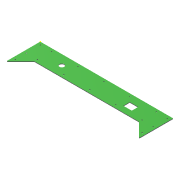
# Autodesk Inventor part: Acrylic Front Panel - No Graphics
Saved by Autodesk Inventor 2017 (Build 210142000, 142)
## iProperties
Created: 2016-07-11
Part Number: Acrylic Front Panel - No Graphics
Material: Generic
Document SubType Name: Modeling
Designer: joshm
Density: 1 g/cm^3
Appearance: Default
Author: joshm
Autodesk Inventor part; units mm, degrees
(part 1 of 2)
ref_plane "YZ Plane" through (0, 0, 0) normal (1, 0, 0) x (0, 1, 0)
ref_plane "XZ Plane" through (0, 0, 0) normal (0, 1, 0) x (-1, 0, 0)
ref_plane "XY Plane" through (0, 0, 0) normal (0, 0, 1) x (1, 0, 0)
sketch "Sketch1" plane through (0, 0, 0) normal (0, 0, 1) x (1, 0, 0)
  line L0 (659.9602, -164.404) -> (660, -164)
  line L1 (660, -164) -> (660, 0)
  line L2 (660, 0) -> (0, 0)
  line L3 (0, 0) -> (0, -164)
  line L4 (0, -164) -> (0.0398, -164.404)
  line L5 (0.0398, -164.404) -> (0.1577, -164.7926)
  line L6 (0.1577, -164.7926) -> (0.349, -165.1506)
  line L7 (0.349, -165.1506) -> (0.6066, -165.4645)
  line L8 (0.6066, -165.4645) -> (0.9204, -165.722)
  line L9 (0.9204, -165.722) -> (1.2785, -165.9134)
  line L10 (1.2785, -165.9134) -> (1.667, -166.0313)
  line L11 (1.667, -166.0313) -> (2.0711, -166.0711)
  line L12 (2.0711, -166.0711) -> (2.4751, -166.0313)
  line L13 (2.4751, -166.0313) -> (2.8636, -165.9134)
  line L14 (2.8636, -165.9134) -> (3.2217, -165.722)
  line L15 (3.2217, -165.722) -> (3.5355, -165.4645)
  line L16 (3.5355, -165.4645) -> (70, -99)
  line L17 (70, -99) -> (590, -99)
  line L18 (590, -99) -> (656.4645, -165.4645)
  line L19 (656.4645, -165.4645) -> (656.7783, -165.722)
  line L20 (656.7783, -165.722) -> (657.1364, -165.9134)
  line L21 (657.1364, -165.9134) -> (657.5249, -166.0313)
  line L22 (657.5249, -166.0313) -> (657.9289, -166.0711)
  line L23 (657.9289, -166.0711) -> (658.333, -166.0313)
  line L24 (658.333, -166.0313) -> (658.7215, -165.9134)
  line L25 (658.7215, -165.9134) -> (659.0796, -165.722)
  line L26 (659.0796, -165.722) -> (659.3934, -165.4645)
  line L27 (659.3934, -165.4645) -> (659.651, -165.1506)
  line L28 (659.651, -165.1506) -> (659.8423, -164.7926)
  line L29 (659.8423, -164.7926) -> (659.9602, -164.404)
  line L30 (590.6522, -86.4341) -> (590, -86.52)
  line L31 (590, -86.52) -> (589.3478, -86.4341)
  line L32 (589.3478, -86.4341) -> (588.74, -86.1824)
  line L33 (588.74, -86.1824) -> (588.2181, -85.7819)
  line L34 (588.2181, -85.7819) -> (587.8176, -85.26)
  line L35 (587.8176, -85.26) -> (587.5659, -84.6522)
  line L36 (587.5659, -84.6522) -> (587.48, -84)
  line L37 (587.48, -84) -> (587.5659, -83.3478)
  line L38 (587.5659, -83.3478) -> (587.8176, -82.74)
  line L39 (587.8176, -82.74) -> (588.2181, -82.2181)
  line L40 (588.2181, -82.2181) -> (588.74, -81.8176)
  line L41 (588.74, -81.8176) -> (589.3478, -81.5659)
  line L42 (589.3478, -81.5659) -> (590, -81.48)
  line L43 (590, -81.48) -> (590.6522, -81.5659)
  line L44 (590.6522, -81.5659) -> (591.26, -81.8176)
  line L45 (591.26, -81.8176) -> (591.7819, -82.2181)
  line L46 (591.7819, -82.2181) -> (592.1824, -82.74)
  line L47 (592.1824, -82.74) -> (592.4341, -83.3478)
  line L48 (592.4341, -83.3478) -> (592.52, -84)
  line L49 (592.52, -84) -> (592.4341, -84.6522)
  line L50 (592.4341, -84.6522) -> (592.1824, -85.26)
  line L51 (592.1824, -85.26) -> (591.7819, -85.7819)
  line L52 (591.7819, -85.7819) -> (591.26, -86.1824)
  line L53 (591.26, -86.1824) -> (590.6522, -86.4341)
  line L54 (457.69, -86.1824) -> (457.1681, -85.7819)
  line L55 (457.1681, -85.7819) -> (456.7676, -85.26)
  line L56 (456.7676, -85.26) -> (456.5159, -84.6522)
  line L57 (456.5159, -84.6522) -> (456.43, -84)
  line L58 (456.43, -84) -> (456.5159, -83.3478)
  line L59 (456.5159, -83.3478) -> (456.7676, -82.74)
  line L60 (456.7676, -82.74) -> (457.1681, -82.2181)
  line L61 (457.1681, -82.2181) -> (457.69, -81.8176)
  line L62 (457.69, -81.8176) -> (458.2978, -81.5659)
  line L63 (458.2978, -81.5659) -> (458.95, -81.48)
  line L64 (458.95, -81.48) -> (459.6022, -81.5659)
  line L65 (459.6022, -81.5659) -> (460.21, -81.8176)
  line L66 (460.21, -81.8176) -> (460.7319, -82.2181)
  line L67 (460.7319, -82.2181) -> (461.1324, -82.74)
  line L68 (461.1324, -82.74) -> (461.3841, -83.3478)
  line L69 (461.3841, -83.3478) -> (461.47, -84)
  line L70 (461.47, -84) -> (461.3841, -84.6522)
  line L71 (461.3841, -84.6522) -> (461.1324, -85.26)
  line L72 (461.1324, -85.26) -> (460.7319, -85.7819)
  line L73 (460.7319, -85.7819) -> (460.21, -86.1824)
  line L74 (460.21, -86.1824) -> (459.6022, -86.4341)
  line L75 (459.6022, -86.4341) -> (458.95, -86.52)
  line L76 (458.95, -86.52) -> (458.2978, -86.4341)
  line L77 (458.2978, -86.4341) -> (457.69, -86.1824)
  line L78 (645.6522, -86.4341) -> (645, -86.52)
  line L79 (645, -86.52) -> (644.3478, -86.4341)
  line L80 (644.3478, -86.4341) -> (643.74, -86.1824)
  line L81 (643.74, -86.1824) -> (643.2181, -85.7819)
  line L82 (643.2181, -85.7819) -> (642.8176, -85.26)
  line L83 (642.8176, -85.26) -> (642.5659, -84.6522)
  line L84 (642.5659, -84.6522) -> (642.48, -84)
  line L85 (642.48, -84) -> (642.5659, -83.3478)
  line L86 (642.5659, -83.3478) -> (642.8176, -82.74)
  line L87 (642.8176, -82.74) -> (643.2181, -82.2181)
  line L88 (643.2181, -82.2181) -> (643.74, -81.8176)
  line L89 (643.74, -81.8176) -> (644.3478, -81.5659)
  line L90 (644.3478, -81.5659) -> (645, -81.48)
  line L91 (645, -81.48) -> (645.6522, -81.5659)
  line L92 (645.6522, -81.5659) -> (646.26, -81.8176)
  line L93 (646.26, -81.8176) -> (646.7819, -82.2181)
  line L94 (646.7819, -82.2181) -> (647.1824, -82.74)
  line L95 (647.1824, -82.74) -> (647.4341, -83.3478)
  line L96 (647.4341, -83.3478) -> (647.52, -84)
  line L97 (647.52, -84) -> (647.4341, -84.6522)
  line L98 (647.4341, -84.6522) -> (647.1824, -85.26)
  line L99 (647.1824, -85.26) -> (646.7819, -85.7819)
  line L100 (646.7819, -85.7819) -> (646.26, -86.1824)
  line L101 (646.26, -86.1824) -> (645.6522, -86.4341)
  line L102 (16.7819, -85.7819) -> (16.26, -86.1824)
  line L103 (16.26, -86.1824) -> (15.6522, -86.4341)
  line L104 (15.6522, -86.4341) -> (15, -86.52)
  line L105 (15, -86.52) -> (14.3478, -86.4341)
  line L106 (14.3478, -86.4341) -> (13.74, -86.1824)
  line L107 (13.74, -86.1824) -> (13.2181, -85.7819)
  line L108 (13.2181, -85.7819) -> (12.8176, -85.26)
  line L109 (12.8176, -85.26) -> (12.5659, -84.6522)
  line L110 (12.5659, -84.6522) -> (12.48, -84)
  line L111 (12.48, -84) -> (12.5659, -83.3478)
  line L112 (12.5659, -83.3478) -> (12.8176, -82.74)
  line L113 (12.8176, -82.74) -> (13.2181, -82.2181)
  line L114 (13.2181, -82.2181) -> (13.74, -81.8176)
  line L115 (13.74, -81.8176) -> (14.3478, -81.5659)
  line L116 (14.3478, -81.5659) -> (15, -81.48)
  line L117 (15, -81.48) -> (15.6522, -81.5659)
  line L118 (15.6522, -81.5659) -> (16.26, -81.8176)
  line L119 (16.26, -81.8176) -> (16.7819, -82.2181)
  line L120 (16.7819, -82.2181) -> (17.1824, -82.74)
  line L121 (17.1824, -82.74) -> (17.4341, -83.3478)
  line L122 (17.4341, -83.3478) -> (17.52, -84)
  line L123 (17.52, -84) -> (17.4341, -84.6522)
  line L124 (17.4341, -84.6522) -> (17.1824, -85.26)
  line L125 (17.1824, -85.26) -> (16.7819, -85.7819)
  line L126 (198.8676, -85.26) -> (198.6159, -84.6522)
  line L127 (198.6159, -84.6522) -> (198.53, -84)
  line L128 (198.53, -84) -> (198.6159, -83.3478)
  line L129 (198.6159, -83.3478) -> (198.8676, -82.74)
  line L130 (198.8676, -82.74) -> (199.2681, -82.2181)
  line L131 (199.2681, -82.2181) -> (199.79, -81.8176)
  line L132 (199.79, -81.8176) -> (200.3978, -81.5659)
  line L133 (200.3978, -81.5659) -> (201.05, -81.48)
  line L134 (201.05, -81.48) -> (201.7022, -81.5659)
  line L135 (201.7022, -81.5659) -> (202.31, -81.8176)
  line L136 (202.31, -81.8176) -> (202.8319, -82.2181)
  line L137 (202.8319, -82.2181) -> (203.2324, -82.74)
  line L138 (203.2324, -82.74) -> (203.4841, -83.3478)
  line L139 (203.4841, -83.3478) -> (203.57, -84)
  line L140 (203.57, -84) -> (203.4841, -84.6522)
  line L141 (203.4841, -84.6522) -> (203.2324, -85.26)
  line L142 (203.2324, -85.26) -> (202.8319, -85.7819)
  line L143 (202.8319, -85.7819) -> (202.31, -86.1824)
  line L144 (202.31, -86.1824) -> (201.7022, -86.4341)
  line L145 (201.7022, -86.4341) -> (201.05, -86.52)
  line L146 (201.05, -86.52) -> (200.3978, -86.4341)
  line L147 (200.3978, -86.4341) -> (199.79, -86.1824)
  line L148 (199.79, -86.1824) -> (199.2681, -85.7819)
  line L149 (199.2681, -85.7819) -> (198.8676, -85.26)
  line L150 (16.7819, -140.7819) -> (16.26, -141.1824)
  line L151 (16.26, -141.1824) -> (15.6522, -141.4341)
  line L152 (15.6522, -141.4341) -> (15, -141.52)
  line L153 (15, -141.52) -> (14.3478, -141.4341)
  line L154 (14.3478, -141.4341) -> (13.74, -141.1824)
  line L155 (13.74, -141.1824) -> (13.2181, -140.7819)
  line L156 (13.2181, -140.7819) -> (12.8176, -140.26)
  line L157 (12.8176, -140.26) -> (12.5659, -139.6522)
  line L158 (12.5659, -139.6522) -> (12.48, -139)
  line L159 (12.48, -139) -> (12.5659, -138.3478)
  line L160 (12.5659, -138.3478) -> (12.8176, -137.74)
  line L161 (12.8176, -137.74) -> (13.2181, -137.2181)
  line L162 (13.2181, -137.2181) -> (13.74, -136.8176)
  line L163 (13.74, -136.8176) -> (14.3478, -136.5659)
  line L164 (14.3478, -136.5659) -> (15, -136.48)
  line L165 (15, -136.48) -> (15.6522, -136.5659)
  line L166 (15.6522, -136.5659) -> (16.26, -136.8176)
  line L167 (16.26, -136.8176) -> (16.7819, -137.2181)
  line L168 (16.7819, -137.2181) -> (17.1824, -137.74)
  line L169 (17.1824, -137.74) -> (17.4341, -138.3478)
  line L170 (17.4341, -138.3478) -> (17.52, -139)
  line L171 (17.52, -139) -> (17.4341, -139.6522)
  line L172 (17.4341, -139.6522) -> (17.1824, -140.26)
  line L173 (17.1824, -140.26) -> (16.7819, -140.7819)
  line L174 (69.3478, -16.4341) -> (68.74, -16.1824)
  line L175 (68.74, -16.1824) -> (68.2181, -15.7819)
  line L176 (68.2181, -15.7819) -> (67.8176, -15.26)
  line L177 (67.8176, -15.26) -> (67.5659, -14.6522)
  line L178 (67.5659, -14.6522) -> (67.48, -14)
  line L179 (67.48, -14) -> (67.5659, -13.3478)
  line L180 (67.5659, -13.3478) -> (67.8176, -12.74)
  line L181 (67.8176, -12.74) -> (68.2181, -12.2181)
  line L182 (68.2181, -12.2181) -> (68.74, -11.8176)
  line L183 (68.74, -11.8176) -> (69.3478, -11.5659)
  line L184 (69.3478, -11.5659) -> (70, -11.48)
  line L185 (70, -11.48) -> (70.6522, -11.5659)
  line L186 (70.6522, -11.5659) -> (71.26, -11.8176)
  line L187 (71.26, -11.8176) -> (71.7819, -12.2181)
  line L188 (71.7819, -12.2181) -> (72.1824, -12.74)
  line L189 (72.1824, -12.74) -> (72.4341, -13.3478)
  line L190 (72.4341, -13.3478) -> (72.52, -14)
  line L191 (72.52, -14) -> (72.4341, -14.6522)
  line L192 (72.4341, -14.6522) -> (72.1824, -15.26)
  line L193 (72.1824, -15.26) -> (71.7819, -15.7819)
  line L194 (71.7819, -15.7819) -> (71.26, -16.1824)
  line L195 (71.26, -16.1824) -> (70.6522, -16.4341)
  line L196 (70.6522, -16.4341) -> (70, -16.52)
  line L197 (70, -16.52) -> (69.3478, -16.4341)
  line L198 (15.6522, -16.4341) -> (15, -16.52)
  line L199 (15, -16.52) -> (14.3478, -16.4341)
  line L200 (14.3478, -16.4341) -> (13.74, -16.1824)
  line L201 (13.74, -16.1824) -> (13.2181, -15.7819)
  line L202 (13.2181, -15.7819) -> (12.8176, -15.26)
  line L203 (12.8176, -15.26) -> (12.5659, -14.6522)
  line L204 (12.5659, -14.6522) -> (12.48, -14)
  line L205 (12.48, -14) -> (12.5659, -13.3478)
  line L206 (12.5659, -13.3478) -> (12.8176, -12.74)
  line L207 (12.8176, -12.74) -> (13.2181, -12.2181)
  line L208 (13.2181, -12.2181) -> (13.74, -11.8176)
  line L209 (13.74, -11.8176) -> (14.3478, -11.5659)
  line L210 (14.3478, -11.5659) -> (15, -11.48)
  line L211 (15, -11.48) -> (15.6522, -11.5659)
  line L212 (15.6522, -11.5659) -> (16.26, -11.8176)
  line L213 (16.26, -11.8176) -> (16.7819, -12.2181)
  line L214 (16.7819, -12.2181) -> (17.1824, -12.74)
  line L215 (17.1824, -12.74) -> (17.4341, -13.3478)
  line L216 (17.4341, -13.3478) -> (17.52, -14)
  line L217 (17.52, -14) -> (17.4341, -14.6522)
  line L218 (17.4341, -14.6522) -> (17.1824, -15.26)
  line L219 (17.1824, -15.26) -> (16.7819, -15.7819)
  line L220 (16.7819, -15.7819) -> (16.26, -16.1824)
  line L221 (16.26, -16.1824) -> (15.6522, -16.4341)
  line L222 (201.7022, -16.4341) -> (201.05, -16.52)
  line L223 (201.05, -16.52) -> (200.3978, -16.4341)
  line L224 (200.3978, -16.4341) -> (199.79, -16.1824)
  line L225 (199.79, -16.1824) -> (199.2681, -15.7819)
  line L226 (199.2681, -15.7819) -> (198.8676, -15.26)
  line L227 (198.8676, -15.26) -> (198.6159, -14.6522)
  line L228 (198.6159, -14.6522) -> (198.53, -14)
  line L229 (198.53, -14) -> (198.6159, -13.3478)
  line L230 (198.6159, -13.3478) -> (198.8676, -12.74)
  line L231 (198.8676, -12.74) -> (199.2681, -12.2181)
  line L232 (199.2681, -12.2181) -> (199.79, -11.8176)
  line L233 (199.79, -11.8176) -> (200.3978, -11.5659)
  line L234 (200.3978, -11.5659) -> (201.05, -11.48)
  line L235 (201.05, -11.48) -> (201.7022, -11.5659)
  line L236 (201.7022, -11.5659) -> (202.31, -11.8176)
  line L237 (202.31, -11.8176) -> (202.8319, -12.2181)
  line L238 (202.8319, -12.2181) -> (203.2324, -12.74)
  line L239 (203.2324, -12.74) -> (203.4841, -13.3478)
  line L240 (203.4841, -13.3478) -> (203.57, -14)
  line L241 (203.57, -14) -> (203.4841, -14.6522)
  line L242 (203.4841, -14.6522) -> (203.2324, -15.26)
  line L243 (203.2324, -15.26) -> (202.8319, -15.7819)
  line L244 (202.8319, -15.7819) -> (202.31, -16.1824)
  line L245 (202.31, -16.1824) -> (201.7022, -16.4341)
  line L246 (330.6522, -16.4341) -> (330, -16.52)
  line L247 (330, -16.52) -> (329.3478, -16.4341)
  line L248 (329.3478, -16.4341) -> (328.74, -16.1824)
  line L249 (328.74, -16.1824) -> (328.2181, -15.7819)
  line L250 (328.2181, -15.7819) -> (327.8176, -15.26)
  line L251 (327.8176, -15.26) -> (327.5659, -14.6522)
  line L252 (327.5659, -14.6522) -> (327.48, -14)
  line L253 (327.48, -14) -> (327.5659, -13.3478)
  line L254 (327.5659, -13.3478) -> (327.8176, -12.74)
  line L255 (327.8176, -12.74) -> (328.2181, -12.2181)
  line L256 (328.2181, -12.2181) -> (328.74, -11.8176)
  line L257 (328.74, -11.8176) -> (329.3478, -11.5659)
  line L258 (329.3478, -11.5659) -> (330, -11.48)
  line L259 (330, -11.48) -> (330.6522, -11.5659)
  line L260 (330.6522, -11.5659) -> (331.26, -11.8176)
  line L261 (331.26, -11.8176) -> (331.7819, -12.2181)
  line L262 (331.7819, -12.2181) -> (332.1824, -12.74)
  line L263 (332.1824, -12.74) -> (332.4341, -13.3478)
  line L264 (332.4341, -13.3478) -> (332.52, -14)
  line L265 (332.52, -14) -> (332.4341, -14.6522)
  line L266 (332.4341, -14.6522) -> (332.1824, -15.26)
  line L267 (332.1824, -15.26) -> (331.7819, -15.7819)
  line L268 (331.7819, -15.7819) -> (331.26, -16.1824)
  line L269 (331.26, -16.1824) -> (330.6522, -16.4341)
  line L270 (644.3478, -16.4341) -> (643.74, -16.1824)
  line L271 (643.74, -16.1824) -> (643.2181, -15.7819)
  line L272 (643.2181, -15.7819) -> (642.8176, -15.26)
  line L273 (642.8176, -15.26) -> (642.5659, -14.6522)
  line L274 (642.5659, -14.6522) -> (642.48, -14)
  line L275 (642.48, -14) -> (642.5659, -13.3478)
  line L276 (642.5659, -13.3478) -> (642.8176, -12.74)
  line L277 (642.8176, -12.74) -> (643.2181, -12.2181)
  line L278 (643.2181, -12.2181) -> (643.74, -11.8176)
  line L279 (643.74, -11.8176) -> (644.3478, -11.5659)
  line L280 (644.3478, -11.5659) -> (645, -11.48)
  line L281 (645, -11.48) -> (645.6522, -11.5659)
  line L282 (645.6522, -11.5659) -> (646.26, -11.8176)
  line L283 (646.26, -11.8176) -> (646.7819, -12.2181)
  line L284 (646.7819, -12.2181) -> (647.1824, -12.74)
  line L285 (647.1824, -12.74) -> (647.4341, -13.3478)
  line L286 (647.4341, -13.3478) -> (647.52, -14)
  line L287 (647.52, -14) -> (647.4341, -14.6522)
  line L288 (647.4341, -14.6522) -> (647.1824, -15.26)
  line L289 (647.1824, -15.26) -> (646.7819, -15.7819)
  line L290 (646.7819, -15.7819) -> (646.26, -16.1824)
  line L291 (646.26, -16.1824) -> (645.6522, -16.4341)
  line L292 (645.6522, -16.4341) -> (645, -16.52)
  line L293 (645, -16.52) -> (644.3478, -16.4341)
  line L294 (459.6022, -16.4341) -> (458.95, -16.52)
  line L295 (458.95, -16.52) -> (458.2978, -16.4341)
  line L296 (458.2978, -16.4341) -> (457.69, -16.1824)
  line L297 (457.69, -16.1824) -> (457.1681, -15.7819)
  line L298 (457.1681, -15.7819) -> (456.7676, -15.26)
  line L299 (456.7676, -15.26) -> (456.5159, -14.6522)
  line L300 (456.5159, -14.6522) -> (456.43, -14)
  line L301 (456.43, -14) -> (456.5159, -13.3478)
  line L302 (456.5159, -13.3478) -> (456.7676, -12.74)
  line L303 (456.7676, -12.74) -> (457.1681, -12.2181)
  line L304 (457.1681, -12.2181) -> (457.69, -11.8176)
  line L305 (457.69, -11.8176) -> (458.2978, -11.5659)
  line L306 (458.2978, -11.5659) -> (458.95, -11.48)
  line L307 (458.95, -11.48) -> (459.6022, -11.5659)
  line L308 (459.6022, -11.5659) -> (460.21, -11.8176)
  line L309 (460.21, -11.8176) -> (460.7319, -12.2181)
  line L310 (460.7319, -12.2181) -> (461.1324, -12.74)
  line L311 (461.1324, -12.74) -> (461.3841, -13.3478)
  line L312 (461.3841, -13.3478) -> (461.47, -14)
  line L313 (461.47, -14) -> (461.3841, -14.6522)
  line L314 (461.3841, -14.6522) -> (461.1324, -15.26)
  line L315 (461.1324, -15.26) -> (460.7319, -15.7819)
  line L316 (460.7319, -15.7819) -> (460.21, -16.1824)
  line L317 (460.21, -16.1824) -> (459.6022, -16.4341)
  line L318 (591.26, -16.1824) -> (590.6522, -16.4341)
  line L319 (590.6522, -16.4341) -> (590, -16.52)
  line L320 (590, -16.52) -> (589.3478, -16.4341)
  line L321 (589.3478, -16.4341) -> (588.74, -16.1824)
  line L322 (588.74, -16.1824) -> (588.2181, -15.7819)
  line L323 (588.2181, -15.7819) -> (587.8176, -15.26)
  line L324 (587.8176, -15.26) -> (587.5659, -14.6522)
  line L325 (587.5659, -14.6522) -> (587.48, -14)
  line L326 (587.48, -14) -> (587.5659, -13.3478)
  line L327 (587.5659, -13.3478) -> (587.8176, -12.74)
  line L328 (587.8176, -12.74) -> (588.2181, -12.2181)
  line L329 (588.2181, -12.2181) -> (588.74, -11.8176)
  line L330 (588.74, -11.8176) -> (589.3478, -11.5659)
  line L331 (589.3478, -11.5659) -> (590, -11.48)
  line L332 (590, -11.48) -> (590.6522, -11.5659)
  line L333 (590.6522, -11.5659) -> (591.26, -11.8176)
  line L334 (591.26, -11.8176) -> (591.7819, -12.2181)
  line L335 (591.7819, -12.2181) -> (592.1824, -12.74)
  line L336 (592.1824, -12.74) -> (592.4341, -13.3478)
  line L337 (592.4341, -13.3478) -> (592.52, -14)
  line L338 (592.52, -14) -> (592.4341, -14.6522)
  line L339 (592.4341, -14.6522) -> (592.1824, -15.26)
  line L340 (592.1824, -15.26) -> (591.7819, -15.7819)
  line L341 (591.7819, -15.7819) -> (591.26, -16.1824)
  line L342 (524.1472, -37.6363) -> (524.1472, -69.6363)
  line L343 (524.1472, -69.6363) -> (482.1472, -69.6363)
  line L344 (482.1472, -69.6363) -> (482.1472, -37.6363)
  line L345 (482.1472, -37.6363) -> (524.1472, -37.6363)
  line L346 (153.0236, -60.1081) -> (150.25, -58.9593)
  line L347 (150.25, -58.9593) -> (147.8683, -57.1317)
  line L348 (147.8683, -57.1317) -> (146.0407, -54.75)
  line L349 (146.0407, -54.75) -> (144.8919, -51.9764)
  line L350 (144.8919, -51.9764) -> (144.5, -49)
  line L351 (144.5, -49) -> (144.8919, -46.0236)
  line L352 (144.8919, -46.0236) -> (146.0407, -43.25)
  line L353 (146.0407, -43.25) -> (147.8683, -40.8683)
  line L354 (147.8683, -40.8683) -> (150.25, -39.0407)
  line L355 (150.25, -39.0407) -> (153.0236, -37.8919)
  line L356 (153.0236, -37.8919) -> (156, -37.5)
  line L357 (156, -37.5) -> (158.9764, -37.8919)
  line L358 (158.9764, -37.8919) -> (161.75, -39.0407)
  line L359 (161.75, -39.0407) -> (164.1317, -40.8683)
  line L360 (164.1317, -40.8683) -> (165.9593, -43.25)
  line L361 (165.9593, -43.25) -> (167.1081, -46.0236)
  line L362 (167.1081, -46.0236) -> (167.5, -49)
  line L363 (167.5, -49) -> (167.1081, -51.9764)
  line L364 (167.1081, -51.9764) -> (165.9593, -54.75)
  line L365 (165.9593, -54.75) -> (164.1317, -57.1317)
  line L366 (164.1317, -57.1317) -> (161.75, -58.9593)
  line L367 (161.75, -58.9593) -> (158.9764, -60.1081)
  line L368 (158.9764, -60.1081) -> (156, -60.5)
  line L369 (156, -60.5) -> (153.0236, -60.1081)
  line L370 (330.6522, -86.4341) -> (330, -86.52)
  line L371 (330, -86.52) -> (329.3478, -86.4341)
  line L372 (329.3478, -86.4341) -> (328.74, -86.1824)
  line L373 (328.74, -86.1824) -> (328.2181, -85.7819)
  line L374 (328.2181, -85.7819) -> (327.8176, -85.26)
  line L375 (327.8176, -85.26) -> (327.5659, -84.6522)
  line L376 (327.5659, -84.6522) -> (327.48, -84)
  line L377 (327.48, -84) -> (327.5659, -83.3478)
  line L378 (327.5659, -83.3478) -> (327.8176, -82.74)
  line L379 (327.8176, -82.74) -> (328.2181, -82.2181)
  line L380 (328.2181, -82.2181) -> (328.74, -81.8176)
  line L381 (328.74, -81.8176) -> (329.3478, -81.5659)
  line L382 (329.3478, -81.5659) -> (330, -81.48)
  line L383 (330, -81.48) -> (330.6522, -81.5659)
  line L384 (330.6522, -81.5659) -> (331.26, -81.8176)
  line L385 (331.26, -81.8176) -> (331.7819, -82.2181)
  line L386 (331.7819, -82.2181) -> (332.1824, -82.74)
  line L387 (332.1824, -82.74) -> (332.4341, -83.3478)
  line L388 (332.4341, -83.3478) -> (332.52, -84)
  line L389 (332.52, -84) -> (332.4341, -84.6522)
  line L390 (332.4341, -84.6522) -> (332.1824, -85.26)
  line L391 (332.1824, -85.26) -> (331.7819, -85.7819)
  line L392 (331.7819, -85.7819) -> (331.26, -86.1824)
  line L393 (331.26, -86.1824) -> (330.6522, -86.4341)
  line L394 (69.3478, -86.4341) -> (68.74, -86.1824)
  line L395 (68.74, -86.1824) -> (68.2181, -85.7819)
  line L396 (68.2181, -85.7819) -> (67.8176, -85.26)
  line L397 (67.8176, -85.26) -> (67.5659, -84.6522)
  line L398 (67.5659, -84.6522) -> (67.48, -84)
  line L399 (67.48, -84) -> (67.5659, -83.3478)
  line L400 (67.5659, -83.3478) -> (67.8176, -82.74)
  line L401 (67.8176, -82.74) -> (68.2181, -82.2181)
  line L402 (68.2181, -82.2181) -> (68.74, -81.8176)
  line L403 (68.74, -81.8176) -> (69.3478, -81.5659)
  line L404 (69.3478, -81.5659) -> (70, -81.48)
  line L405 (70, -81.48) -> (70.6522, -81.5659)
  line L406 (70.6522, -81.5659) -> (71.26, -81.8176)
  line L407 (71.26, -81.8176) -> (71.7819, -82.2181)
  line L408 (71.7819, -82.2181) -> (72.1824, -82.74)
  line L409 (72.1824, -82.74) -> (72.4341, -83.3478)
  line L410 (72.4341, -83.3478) -> (72.52, -84)
  line L411 (72.52, -84) -> (72.4341, -84.6522)
  line L412 (72.4341, -84.6522) -> (72.1824, -85.26)
  line L413 (72.1824, -85.26) -> (71.7819, -85.7819)
  line L414 (71.7819, -85.7819) -> (71.26, -86.1824)
  line L415 (71.26, -86.1824) -> (70.6522, -86.4341)
  line L416 (70.6522, -86.4341) -> (70, -86.52)
  line L417 (70, -86.52) -> (69.3478, -86.4341)
  line L418 (645.6522, -141.4544) -> (645, -141.541)
  line L419 (645, -141.541) -> (644.3478, -141.4544)
  line L420 (644.3478, -141.4544) -> (643.74, -141.2006)
  line L421 (643.74, -141.2006) -> (643.2181, -140.7968)
  line L422 (643.2181, -140.7968) -> (642.8176, -140.2705)
  line L423 (642.8176, -140.2705) -> (642.5659, -139.6577)
  line L424 (642.5659, -139.6577) -> (642.48, -139)
  line L425 (642.48, -139) -> (642.5659, -138.3423)
  line L426 (642.5659, -138.3423) -> (642.8176, -137.7295)
  line L427 (642.8176, -137.7295) -> (643.2181, -137.2032)
  line L428 (643.2181, -137.2032) -> (643.74, -136.7994)
  line L429 (643.74, -136.7994) -> (644.3478, -136.5456)
  line L430 (644.3478, -136.5456) -> (645, -136.459)
  line L431 (645, -136.459) -> (645.6522, -136.5456)
  line L432 (645.6522, -136.5456) -> (646.26, -136.7994)
  line L433 (646.26, -136.7994) -> (646.7819, -137.2032)
  line L434 (646.7819, -137.2032) -> (647.1824, -137.7295)
  line L435 (647.1824, -137.7295) -> (647.4341, -138.3423)
  line L436 (647.4341, -138.3423) -> (647.52, -139)
  line L437 (647.52, -139) -> (647.4341, -139.6577)
  line L438 (647.4341, -139.6577) -> (647.1824, -140.2705)
  line L439 (647.1824, -140.2705) -> (646.7819, -140.7968)
  line L440 (646.7819, -140.7968) -> (646.26, -141.2006)
  line L441 (646.26, -141.2006) -> (645.6522, -141.4544)
  constraints: 884 end point, 1 coincident
extrude "Extrusion1" add sketch "Sketch1" along normal blind 3
sketch "Sketch2" plane through (0, 0, 3) normal (0, 0, 1) x (1, 0, 0)
  line L0 (482.1472, -69.6363) -> (482.1472, -37.6363) projected
  line L1 (482.1472, -37.6363) -> (524.1472, -37.6363) projected
  line L2 (524.1472, -37.6363) -> (524.1472, -69.6363) projected
  line L3 (524.1472, -69.6363) -> (482.1472, -69.6363) projected
  line L4 (147.8683, -57.1317) -> (146.0407, -54.75) projected
  line L5 (146.0407, -54.75) -> (144.8919, -51.9764) projected
  line L6 (144.8919, -51.9764) -> (144.5, -49) projected
  line L7 (144.5, -49) -> (144.8919, -46.0236) projected
  line L8 (144.8919, -46.0236) -> (146.0407, -43.25) projected
  line L9 (146.0407, -43.25) -> (147.8683, -40.8683) projected
  line L10 (147.8683, -40.8683) -> (150.25, -39.0407) projected
  line L11 (150.25, -39.0407) -> (153.0236, -37.8919) projected
  line L12 (153.0236, -37.8919) -> (156, -37.5) projected
  line L13 (156, -37.5) -> (158.9764, -37.8919) projected
  line L14 (158.9764, -37.8919) -> (161.75, -39.0407) projected
  line L15 (161.75, -39.0407) -> (164.1317, -40.8683) projected
  line L16 (164.1317, -40.8683) -> (165.9593, -43.25) projected
  line L17 (165.9593, -43.25) -> (167.1081, -46.0236) projected
  line L18 (167.1081, -46.0236) -> (167.5, -49) projected
  line L19 (167.5, -49) -> (167.1081, -51.9764) projected
  line L20 (167.1081, -51.9764) -> (165.9593, -54.75) projected
  line L21 (165.9593, -54.75) -> (164.1317, -57.1317) projected
  line L22 (164.1317, -57.1317) -> (161.75, -58.9593) projected
  line L23 (161.75, -58.9593) -> (158.9764, -60.1081) projected
  line L24 (158.9764, -60.1081) -> (156, -60.5) projected
  line L25 (156, -60.5) -> (153.0236, -60.1081) projected
  line L26 (153.0236, -60.1081) -> (150.25, -58.9593) projected
  line L27 (150.25, -58.9593) -> (147.8683, -57.1317) projected
  line L28 (644.3478, -141.4544) -> (643.74, -141.2006) projected
  line L29 (643.74, -141.2006) -> (643.2181, -140.7968) projected
  line L30 (643.2181, -140.7968) -> (642.8176, -140.2705) projected
  line L31 (642.8176, -140.2705) -> (642.5659, -139.6577) projected
  line L32 (642.5659, -139.6577) -> (642.48, -139) projected
  line L33 (642.48, -139) -> (642.5659, -138.3423) projected
  line L34 (642.5659, -138.3423) -> (642.8176, -137.7295) projected
  line L35 (642.8176, -137.7295) -> (643.2181, -137.2032) projected
  line L36 (643.2181, -137.2032) -> (643.74, -136.7994) projected
  line L37 (643.74, -136.7994) -> (644.3478, -136.5456) projected
  line L38 (644.3478, -136.5456) -> (645, -136.459) projected
  line L39 (645, -136.459) -> (645.6522, -136.5456) projected
  line L40 (645.6522, -136.5456) -> (646.26, -136.7994) projected
  line L41 (646.26, -136.7994) -> (646.7819, -137.2032) projected
  line L42 (646.7819, -137.2032) -> (647.1824, -137.7295) projected
  line L43 (647.1824, -137.7295) -> (647.4341, -138.3423) projected
  line L44 (647.4341, -138.3423) -> (647.52, -139) projected
  line L45 (647.52, -139) -> (647.4341, -139.6577) projected
  line L46 (647.4341, -139.6577) -> (647.1824, -140.2705) projected
  line L47 (647.1824, -140.2705) -> (646.7819, -140.7968) projected
  line L48 (646.7819, -140.7968) -> (646.26, -141.2006) projected
  line L49 (646.26, -141.2006) -> (645.6522, -141.4544) projected
  line L50 (645.6522, -141.4544) -> (645, -141.541) projected
  line L51 (645, -141.541) -> (644.3478, -141.4544) projected
  line L52 (68.2181, -85.7819) -> (67.8176, -85.26) projected
  line L53 (67.8176, -85.26) -> (67.5659, -84.6522) projected
  line L54 (67.5659, -84.6522) -> (67.48, -84) projected
  line L55 (67.48, -84) -> (67.5659, -83.3478) projected
  line L56 (67.5659, -83.3478) -> (67.8176, -82.74) projected
  line L57 (67.8176, -82.74) -> (68.2181, -82.2181) projected
  line L58 (68.2181, -82.2181) -> (68.74, -81.8176) projected
  line L59 (68.74, -81.8176) -> (69.3478, -81.5659) projected
  line L60 (69.3478, -81.5659) -> (70, -81.48) projected
  line L61 (70, -81.48) -> (70.6522, -81.5659) projected
  line L62 (70.6522, -81.5659) -> (71.26, -81.8176) projected
  line L63 (71.26, -81.8176) -> (71.7819, -82.2181) projected
  line L64 (71.7819, -82.2181) -> (72.1824, -82.74) projected
  line L65 (72.1824, -82.74) -> (72.4341, -83.3478) projected
  line L66 (72.4341, -83.3478) -> (72.52, -84) projected
  line L67 (72.52, -84) -> (72.4341, -84.6522) projected
  line L68 (72.4341, -84.6522) -> (72.1824, -85.26) projected
  line L69 (72.1824, -85.26) -> (71.7819, -85.7819) projected
  line L70 (71.7819, -85.7819) -> (71.26, -86.1824) projected
  line L71 (71.26, -86.1824) -> (70.6522, -86.4341) projected
  line L72 (70.6522, -86.4341) -> (70, -86.52) projected
  line L73 (70, -86.52) -> (69.3478, -86.4341) projected
  line L74 (69.3478, -86.4341) -> (68.74, -86.1824) projected
  line L75 (68.74, -86.1824) -> (68.2181, -85.7819) projected
  line L76 (329.3478, -86.4341) -> (328.74, -86.1824) projected
  line L77 (328.74, -86.1824) -> (328.2181, -85.7819) projected
  line L78 (328.2181, -85.7819) -> (327.8176, -85.26) projected
  line L79 (327.8176, -85.26) -> (327.5659, -84.6522) projected
  line L80 (327.5659, -84.6522) -> (327.48, -84) projected
  line L81 (327.48, -84) -> (327.5659, -83.3478) projected
  line L82 (327.5659, -83.3478) -> (327.8176, -82.74) projected
  line L83 (327.8176, -82.74) -> (328.2181, -82.2181) projected
  line L84 (328.2181, -82.2181) -> (328.74, -81.8176) projected
  line L85 (328.74, -81.8176) -> (329.3478, -81.5659) projected
  line L86 (329.3478, -81.5659) -> (330, -81.48) projected
  line L87 (330, -81.48) -> (330.6522, -81.5659) projected
  line L88 (330.6522, -81.5659) -> (331.26, -81.8176) projected
  line L89 (331.26, -81.8176) -> (331.7819, -82.2181) projected
  line L90 (331.7819, -82.2181) -> (332.1824, -82.74) projected
  line L91 (332.1824, -82.74) -> (332.4341, -83.3478) projected
  line L92 (332.4341, -83.3478) -> (332.52, -84) projected
  line L93 (332.52, -84) -> (332.4341, -84.6522) projected
  line L94 (332.4341, -84.6522) -> (332.1824, -85.26) projected
  line L95 (332.1824, -85.26) -> (331.7819, -85.7819) projected
  line L96 (331.7819, -85.7819) -> (331.26, -86.1824) projected
  line L97 (331.26, -86.1824) -> (330.6522, -86.4341) projected
  line L98 (330.6522, -86.4341) -> (330, -86.52) projected
  line L99 (330, -86.52) -> (329.3478, -86.4341) projected
  line L100 (590, -16.52) -> (589.3478, -16.4341) projected
  line L101 (589.3478, -16.4341) -> (588.74, -16.1824) projected
  line L102 (588.74, -16.1824) -> (588.2181, -15.7819) projected
  line L103 (588.2181, -15.7819) -> (587.8176, -15.26) projected
  line L104 (587.8176, -15.26) -> (587.5659, -14.6522) projected
  line L105 (587.5659, -14.6522) -> (587.48, -14) projected
  line L106 (587.48, -14) -> (587.5659, -13.3478) projected
  line L107 (587.5659, -13.3478) -> (587.8176, -12.74) projected
  line L108 (587.8176, -12.74) -> (588.2181, -12.2181) projected
  line L109 (588.2181, -12.2181) -> (588.74, -11.8176) projected
  line L110 (588.74, -11.8176) -> (589.3478, -11.5659) projected
  line L111 (589.3478, -11.5659) -> (590, -11.48) projected
  line L112 (590, -11.48) -> (590.6522, -11.5659) projected
  line L113 (590.6522, -11.5659) -> (591.26, -11.8176) projected
  line L114 (591.26, -11.8176) -> (591.7819, -12.2181) projected
  line L115 (591.7819, -12.2181) -> (592.1824, -12.74) projected
  line L116 (592.1824, -12.74) -> (592.4341, -13.3478) projected
  line L117 (592.4341, -13.3478) -> (592.52, -14) projected
  line L118 (592.52, -14) -> (592.4341, -14.6522) projected
  line L119 (592.4341, -14.6522) -> (592.1824, -15.26) projected
  line L120 (592.1824, -15.26) -> (591.7819, -15.7819) projected
  line L121 (591.7819, -15.7819) -> (591.26, -16.1824) projected
  line L122 (591.26, -16.1824) -> (590.6522, -16.4341) projected
  line L123 (590.6522, -16.4341) -> (590, -16.52) projected
  line L124 (458.2978, -16.4341) -> (457.69, -16.1824) projected
  line L125 (457.69, -16.1824) -> (457.1681, -15.7819) projected
  line L126 (457.1681, -15.7819) -> (456.7676, -15.26) projected
  line L127 (456.7676, -15.26) -> (456.5159, -14.6522) projected
  line L128 (456.5159, -14.6522) -> (456.43, -14) projected
  line L129 (456.43, -14) -> (456.5159, -13.3478) projected
  line L130 (456.5159, -13.3478) -> (456.7676, -12.74) projected
  line L131 (456.7676, -12.74) -> (457.1681, -12.2181) projected
  line L132 (457.1681, -12.2181) -> (457.69, -11.8176) projected
  line L133 (457.69, -11.8176) -> (458.2978, -11.5659) projected
  line L134 (458.2978, -11.5659) -> (458.95, -11.48) projected
  line L135 (458.95, -11.48) -> (459.6022, -11.5659) projected
  line L136 (459.6022, -11.5659) -> (460.21, -11.8176) projected
  line L137 (460.21, -11.8176) -> (460.7319, -12.2181) projected
  line L138 (460.7319, -12.2181) -> (461.1324, -12.74) projected
  line L139 (461.1324, -12.74) -> (461.3841, -13.3478) projected
  line L140 (461.3841, -13.3478) -> (461.47, -14) projected
  line L141 (461.47, -14) -> (461.3841, -14.6522) projected
  line L142 (461.3841, -14.6522) -> (461.1324, -15.26) projected
  line L143 (461.1324, -15.26) -> (460.7319, -15.7819) projected
  line L144 (460.7319, -15.7819) -> (460.21, -16.1824) projected
  line L145 (460.21, -16.1824) -> (459.6022, -16.4341) projected
  line L146 (459.6022, -16.4341) -> (458.95, -16.52) projected
  line L147 (458.95, -16.52) -> (458.2978, -16.4341) projected
  line L148 (643.2181, -15.7819) -> (642.8176, -15.26) projected
  line L149 (642.8176, -15.26) -> (642.5659, -14.6522) projected
  line L150 (642.5659, -14.6522) -> (642.48, -14) projected
  line L151 (642.48, -14) -> (642.5659, -13.3478) projected
  line L152 (642.5659, -13.3478) -> (642.8176, -12.74) projected
  line L153 (642.8176, -12.74) -> (643.2181, -12.2181) projected
  line L154 (643.2181, -12.2181) -> (643.74, -11.8176) projected
  line L155 (643.74, -11.8176) -> (644.3478, -11.5659) projected
  line L156 (644.3478, -11.5659) -> (645, -11.48) projected
  line L157 (645, -11.48) -> (645.6522, -11.5659) projected
  line L158 (645.6522, -11.5659) -> (646.26, -11.8176) projected
  line L159 (646.26, -11.8176) -> (646.7819, -12.2181) projected
  line L160 (646.7819, -12.2181) -> (647.1824, -12.74) projected
  line L161 (647.1824, -12.74) -> (647.4341, -13.3478) projected
  line L162 (647.4341, -13.3478) -> (647.52, -14) projected
  line L163 (647.52, -14) -> (647.4341, -14.6522) projected
  line L164 (647.4341, -14.6522) -> (647.1824, -15.26) projected
  line L165 (647.1824, -15.26) -> (646.7819, -15.7819) projected
  line L166 (646.7819, -15.7819) -> (646.26, -16.1824) projected
  line L167 (646.26, -16.1824) -> (645.6522, -16.4341) projected
  line L168 (645.6522, -16.4341) -> (645, -16.52) projected
  line L169 (645, -16.52) -> (644.3478, -16.4341) projected
  line L170 (644.3478, -16.4341) -> (643.74, -16.1824) projected
  line L171 (643.74, -16.1824) -> (643.2181, -15.7819) projected
  line L172 (329.3478, -16.4341) -> (328.74, -16.1824) projected
  line L173 (328.74, -16.1824) -> (328.2181, -15.7819) projected
  line L174 (328.2181, -15.7819) -> (327.8176, -15.26) projected
  line L175 (327.8176, -15.26) -> (327.5659, -14.6522) projected
  line L176 (327.5659, -14.6522) -> (327.48, -14) projected
  line L177 (327.48, -14) -> (327.5659, -13.3478) projected
  line L178 (327.5659, -13.3478) -> (327.8176, -12.74) projected
  line L179 (327.8176, -12.74) -> (328.2181, -12.2181) projected
  line L180 (328.2181, -12.2181) -> (328.74, -11.8176) projected
  line L181 (328.74, -11.8176) -> (329.3478, -11.5659) projected
  line L182 (329.3478, -11.5659) -> (330, -11.48) projected
  line L183 (330, -11.48) -> (330.6522, -11.5659) projected
  line L184 (330.6522, -11.5659) -> (331.26, -11.8176) projected
  line L185 (331.26, -11.8176) -> (331.7819, -12.2181) projected
  line L186 (331.7819, -12.2181) -> (332.1824, -12.74) projected
  line L187 (332.1824, -12.74) -> (332.4341, -13.3478) projected
  line L188 (332.4341, -13.3478) -> (332.52, -14) projected
  line L189 (332.52, -14) -> (332.4341, -14.6522) projected
  line L190 (332.4341, -14.6522) -> (332.1824, -15.26) projected
  line L191 (332.1824, -15.26) -> (331.7819, -15.7819) projected
  line L192 (331.7819, -15.7819) -> (331.26, -16.1824) projected
  line L193 (331.26, -16.1824) -> (330.6522, -16.4341) projected
  line L194 (330.6522, -16.4341) -> (330, -16.52) projected
  line L195 (330, -16.52) -> (329.3478, -16.4341) projected
  line L196 (200.3978, -16.4341) -> (199.79, -16.1824) projected
  line L197 (199.79, -16.1824) -> (199.2681, -15.7819) projected
  line L198 (199.2681, -15.7819) -> (198.8676, -15.26) projected
  line L199 (198.8676, -15.26) -> (198.6159, -14.6522) projected
  line L200 (198.6159, -14.6522) -> (198.53, -14) projected
  line L201 (198.53, -14) -> (198.6159, -13.3478) projected
  line L202 (198.6159, -13.3478) -> (198.8676, -12.74) projected
  line L203 (198.8676, -12.74) -> (199.2681, -12.2181) projected
  line L204 (199.2681, -12.2181) -> (199.79, -11.8176) projected
  line L205 (199.79, -11.8176) -> (200.3978, -11.5659) projected
  line L206 (200.3978, -11.5659) -> (201.05, -11.48) projected
  line L207 (201.05, -11.48) -> (201.7022, -11.5659) projected
  line L208 (201.7022, -11.5659) -> (202.31, -11.8176) projected
  line L209 (202.31, -11.8176) -> (202.8319, -12.2181) projected
  line L210 (202.8319, -12.2181) -> (203.2324, -12.74) projected
  line L211 (203.2324, -12.74) -> (203.4841, -13.3478) projected
  line L212 (203.4841, -13.3478) -> (203.57, -14) projected
  line L213 (203.57, -14) -> (203.4841, -14.6522) projected
  line L214 (203.4841, -14.6522) -> (203.2324, -15.26) projected
  line L215 (203.2324, -15.26) -> (202.8319, -15.7819) projected
  line L216 (202.8319, -15.7819) -> (202.31, -16.1824) projected
  line L217 (202.31, -16.1824) -> (201.7022, -16.4341) projected
  line L218 (201.7022, -16.4341) -> (201.05, -16.52) projected
  line L219 (201.05, -16.52) -> (200.3978, -16.4341) projected
  line L220 (14.3478, -16.4341) -> (13.74, -16.1824) projected
  line L221 (13.74, -16.1824) -> (13.2181, -15.7819) projected
  line L222 (13.2181, -15.7819) -> (12.8176, -15.26) projected
  line L223 (12.8176, -15.26) -> (12.5659, -14.6522) projected
  line L224 (12.5659, -14.6522) -> (12.48, -14) projected
  line L225 (12.48, -14) -> (12.5659, -13.3478) projected
  line L226 (12.5659, -13.3478) -> (12.8176, -12.74) projected
  line L227 (12.8176, -12.74) -> (13.2181, -12.2181) projected
  line L228 (13.2181, -12.2181) -> (13.74, -11.8176) projected
  line L229 (13.74, -11.8176) -> (14.3478, -11.5659) projected
  line L230 (14.3478, -11.5659) -> (15, -11.48) projected
  line L231 (15, -11.48) -> (15.6522, -11.5659) projected
  line L232 (15.6522, -11.5659) -> (16.26, -11.8176) projected
  line L233 (16.26, -11.8176) -> (16.7819, -12.2181) projected
  line L234 (16.7819, -12.2181) -> (17.1824, -12.74) projected
  line L235 (17.1824, -12.74) -> (17.4341, -13.3478) projected
  line L236 (17.4341, -13.3478) -> (17.52, -14) projected
  line L237 (17.52, -14) -> (17.4341, -14.6522) projected
  line L238 (17.4341, -14.6522) -> (17.1824, -15.26) projected
  line L239 (17.1824, -15.26) -> (16.7819, -15.7819) projected
  line L240 (16.7819, -15.7819) -> (16.26, -16.1824) projected
  line L241 (16.26, -16.1824) -> (15.6522, -16.4341) projected
  line L242 (15.6522, -16.4341) -> (15, -16.52) projected
  line L243 (15, -16.52) -> (14.3478, -16.4341) projected
  line L244 (68.2181, -15.7819) -> (67.8176, -15.26) projected
  line L245 (67.8176, -15.26) -> (67.5659, -14.6522) projected
  line L246 (67.5659, -14.6522) -> (67.48, -14) projected
  line L247 (67.48, -14) -> (67.5659, -13.3478) projected
  line L248 (67.5659, -13.3478) -> (67.8176, -12.74) projected
  line L249 (67.8176, -12.74) -> (68.2181, -12.2181) projected
  line L250 (68.2181, -12.2181) -> (68.74, -11.8176) projected
  line L251 (68.74, -11.8176) -> (69.3478, -11.5659) projected
  line L252 (69.3478, -11.5659) -> (70, -11.48) projected
  line L253 (70, -11.48) -> (70.6522, -11.5659) projected
  line L254 (70.6522, -11.5659) -> (71.26, -11.8176) projected
  line L255 (71.26, -11.8176) -> (71.7819, -12.2181) projected
  line L256 (71.7819, -12.2181) -> (72.1824, -12.74) projected
  line L257 (72.1824, -12.74) -> (72.4341, -13.3478) projected
  line L258 (72.4341, -13.3478) -> (72.52, -14) projected
  line L259 (72.52, -14) -> (72.4341, -14.6522) projected
  line L260 (72.4341, -14.6522) -> (72.1824, -15.26) projected
  line L261 (72.1824, -15.26) -> (71.7819, -15.7819) projected
  line L262 (71.7819, -15.7819) -> (71.26, -16.1824) projected
  line L263 (71.26, -16.1824) -> (70.6522, -16.4341) projected
  line L264 (70.6522, -16.4341) -> (70, -16.52) projected
  line L265 (70, -16.52) -> (69.3478, -16.4341) projected
  line L266 (69.3478, -16.4341) -> (68.74, -16.1824) projected
  line L267 (68.74, -16.1824) -> (68.2181, -15.7819) projected
  line L268 (15.6522, -141.4341) -> (15, -141.52) projected
  line L269 (15, -141.52) -> (14.3478, -141.4341) projected
  line L270 (14.3478, -141.4341) -> (13.74, -141.1824) projected
  line L271 (13.74, -141.1824) -> (13.2181, -140.7819) projected
  line L272 (13.2181, -140.7819) -> (12.8176, -140.26) projected
  line L273 (12.8176, -140.26) -> (12.5659, -139.6522) projected
  line L274 (12.5659, -139.6522) -> (12.48, -139) projected
  line L275 (12.48, -139) -> (12.5659, -138.3478) projected
  line L276 (12.5659, -138.3478) -> (12.8176, -137.74) projected
  line L277 (12.8176, -137.74) -> (13.2181, -137.2181) projected
  line L278 (13.2181, -137.2181) -> (13.74, -136.8176) projected
  line L279 (13.74, -136.8176) -> (14.3478, -136.5659) projected
  line L280 (14.3478, -136.5659) -> (15, -136.48) projected
  line L281 (15, -136.48) -> (15.6522, -136.5659) projected
  line L282 (15.6522, -136.5659) -> (16.26, -136.8176) projected
  line L283 (16.26, -136.8176) -> (16.7819, -137.2181) projected
  line L284 (16.7819, -137.2181) -> (17.1824, -137.74) projected
  line L285 (17.1824, -137.74) -> (17.4341, -138.3478) projected
  line L286 (17.4341, -138.3478) -> (17.52, -139) projected
  line L287 (17.52, -139) -> (17.4341, -139.6522) projected
  line L288 (17.4341, -139.6522) -> (17.1824, -140.26) projected
  line L289 (17.1824, -140.26) -> (16.7819, -140.7819) projected
  line L290 (16.7819, -140.7819) -> (16.26, -141.1824) projected
  line L291 (16.26, -141.1824) -> (15.6522, -141.4341) projected
  line L292 (198.53, -84) -> (198.6159, -83.3478) projected
  line L293 (198.6159, -83.3478) -> (198.8676, -82.74) projected
  line L294 (198.8676, -82.74) -> (199.2681, -82.2181) projected
  line L295 (199.2681, -82.2181) -> (199.79, -81.8176) projected
  line L296 (199.79, -81.8176) -> (200.3978, -81.5659) projected
  line L297 (200.3978, -81.5659) -> (201.05, -81.48) projected
  line L298 (201.05, -81.48) -> (201.7022, -81.5659) projected
  line L299 (201.7022, -81.5659) -> (202.31, -81.8176) projected
  line L300 (202.31, -81.8176) -> (202.8319, -82.2181) projected
  line L301 (202.8319, -82.2181) -> (203.2324, -82.74) projected
  line L302 (203.2324, -82.74) -> (203.4841, -83.3478) projected
  line L303 (203.4841, -83.3478) -> (203.57, -84) projected
  line L304 (203.57, -84) -> (203.4841, -84.6522) projected
  line L305 (203.4841, -84.6522) -> (203.2324, -85.26) projected
  line L306 (203.2324, -85.26) -> (202.8319, -85.7819) projected
  line L307 (202.8319, -85.7819) -> (202.31, -86.1824) projected
  line L308 (202.31, -86.1824) -> (201.7022, -86.4341) projected
  line L309 (201.7022, -86.4341) -> (201.05, -86.52) projected
  line L310 (201.05, -86.52) -> (200.3978, -86.4341) projected
  line L311 (200.3978, -86.4341) -> (199.79, -86.1824) projected
  line L312 (199.79, -86.1824) -> (199.2681, -85.7819) projected
  line L313 (199.2681, -85.7819) -> (198.8676, -85.26) projected
  line L314 (198.8676, -85.26) -> (198.6159, -84.6522) projected
  line L315 (198.6159, -84.6522) -> (198.53, -84) projected
  line L316 (15.6522, -86.4341) -> (15, -86.52) projected
  line L317 (15, -86.52) -> (14.3478, -86.4341) projected
  line L318 (14.3478, -86.4341) -> (13.74, -86.1824) projected
  line L319 (13.74, -86.1824) -> (13.2181, -85.7819) projected
  line L320 (13.2181, -85.7819) -> (12.8176, -85.26) projected
  line L321 (12.8176, -85.26) -> (12.5659, -84.6522) projected
  line L322 (12.5659, -84.6522) -> (12.48, -84) projected
  line L323 (12.48, -84) -> (12.5659, -83.3478) projected
  line L324 (12.5659, -83.3478) -> (12.8176, -82.74) projected
  line L325 (12.8176, -82.74) -> (13.2181, -82.2181) projected
  line L326 (13.2181, -82.2181) -> (13.74, -81.8176) projected
  line L327 (13.74, -81.8176) -> (14.3478, -81.5659) projected
  line L328 (14.3478, -81.5659) -> (15, -81.48) projected
  line L329 (15, -81.48) -> (15.6522, -81.5659) projected
  line L330 (15.6522, -81.5659) -> (16.26, -81.8176) projected
  line L331 (16.26, -81.8176) -> (16.7819, -82.2181) projected
  line L332 (16.7819, -82.2181) -> (17.1824, -82.74) projected
  line L333 (17.1824, -82.74) -> (17.4341, -83.3478) projected
  line L334 (17.4341, -83.3478) -> (17.52, -84) projected
  line L335 (17.52, -84) -> (17.4341, -84.6522) projected
  line L336 (17.4341, -84.6522) -> (17.1824, -85.26) projected
  line L337 (17.1824, -85.26) -> (16.7819, -85.7819) projected
  line L338 (16.7819, -85.7819) -> (16.26, -86.1824) projected
  line L339 (16.26, -86.1824) -> (15.6522, -86.4341) projected
  line L340 (644.3478, -86.4341) -> (643.74, -86.1824) projected
  line L341 (643.74, -86.1824) -> (643.2181, -85.7819) projected
  line L342 (643.2181, -85.7819) -> (642.8176, -85.26) projected
  line L343 (642.8176, -85.26) -> (642.5659, -84.6522) projected
  line L344 (642.5659, -84.6522) -> (642.48, -84) projected
  line L345 (642.48, -84) -> (642.5659, -83.3478) projected
  line L346 (642.5659, -83.3478) -> (642.8176, -82.74) projected
  line L347 (642.8176, -82.74) -> (643.2181, -82.2181) projected
  line L348 (643.2181, -82.2181) -> (643.74, -81.8176) projected
  line L349 (643.74, -81.8176) -> (644.3478, -81.5659) projected
  line L350 (644.3478, -81.5659) -> (645, -81.48) projected
  line L351 (645, -81.48) -> (645.6522, -81.5659) projected
  line L352 (645.6522, -81.5659) -> (646.26, -81.8176) projected
  line L353 (646.26, -81.8176) -> (646.7819, -82.2181) projected
  line L354 (646.7819, -82.2181) -> (647.1824, -82.74) projected
  line L355 (647.1824, -82.74) -> (647.4341, -83.3478) projected
  line L356 (647.4341, -83.3478) -> (647.52, -84) projected
  line L357 (647.52, -84) -> (647.4341, -84.6522) projected
  line L358 (647.4341, -84.6522) -> (647.1824, -85.26) projected
  line L359 (647.1824, -85.26) -> (646.7819, -85.7819) projected
  line L360 (646.7819, -85.7819) -> (646.26, -86.1824) projected
  line L361 (646.26, -86.1824) -> (645.6522, -86.4341) projected
  line L362 (645.6522, -86.4341) -> (645, -86.52) projected
  line L363 (645, -86.52) -> (644.3478, -86.4341) projected
  line L364 (456.7676, -85.26) -> (456.5159, -84.6522) projected
  line L365 (456.5159, -84.6522) -> (456.43, -84) projected
  line L366 (456.43, -84) -> (456.5159, -83.3478) projected
  line L367 (456.5159, -83.3478) -> (456.7676, -82.74) projected
  line L368 (456.7676, -82.74) -> (457.1681, -82.2181) projected
  line L369 (457.1681, -82.2181) -> (457.69, -81.8176) projected
  line L370 (457.69, -81.8176) -> (458.2978, -81.5659) projected
  line L371 (458.2978, -81.5659) -> (458.95, -81.48) projected
  line L372 (458.95, -81.48) -> (459.6022, -81.5659) projected
  line L373 (459.6022, -81.5659) -> (460.21, -81.8176) projected
  line L374 (460.21, -81.8176) -> (460.7319, -82.2181) projected
  line L375 (460.7319, -82.2181) -> (461.1324, -82.74) projected
  line L376 (461.1324, -82.74) -> (461.3841, -83.3478) projected
  line L377 (461.3841, -83.3478) -> (461.47, -84) projected
  line L378 (461.47, -84) -> (461.3841, -84.6522) projected
  line L379 (461.3841, -84.6522) -> (461.1324, -85.26) projected
  line L380 (461.1324, -85.26) -> (460.7319, -85.7819) projected
  line L381 (460.7319, -85.7819) -> (460.21, -86.1824) projected
  line L382 (460.21, -86.1824) -> (459.6022, -86.4341) projected
  line L383 (459.6022, -86.4341) -> (458.95, -86.52) projected
  line L384 (458.95, -86.52) -> (458.2978, -86.4341) projected
  line L385 (458.2978, -86.4341) -> (457.69, -86.1824) projected
  line L386 (457.69, -86.1824) -> (457.1681, -85.7819) projected
  line L387 (457.1681, -85.7819) -> (456.7676, -85.26) projected
  line L388 (589.3478, -86.4341) -> (588.74, -86.1824) projected
  line L389 (588.74, -86.1824) -> (588.2181, -85.7819) projected
  line L390 (588.2181, -85.7819) -> (587.8176, -85.26) projected
  line L391 (587.8176, -85.26) -> (587.5659, -84.6522) projected
  line L392 (587.5659, -84.6522) -> (587.48, -84) projected
  line L393 (587.48, -84) -> (587.5659, -83.3478) projected
  line L394 (587.5659, -83.3478) -> (587.8176, -82.74) projected
  line L395 (587.8176, -82.74) -> (588.2181, -82.2181) projected
  line L396 (588.2181, -82.2181) -> (588.74, -81.8176) projected
  line L397 (588.74, -81.8176) -> (589.3478, -81.5659) projected
  line L398 (589.3478, -81.5659) -> (590, -81.48) projected
  line L399 (590, -81.48) -> (590.6522, -81.5659) projected
  line L400 (590.6522, -81.5659) -> (591.26, -81.8176) projected
  line L401 (591.26, -81.8176) -> (591.7819, -82.2181) projected
  line L402 (591.7819, -82.2181) -> (592.1824, -82.74) projected
  line L403 (592.1824, -82.74) -> (592.4341, -83.3478) projected
  line L404 (592.4341, -83.3478) -> (592.52, -84) projected
  line L405 (592.52, -84) -> (592.4341, -84.6522) projected
  line L406 (592.4341, -84.6522) -> (592.1824, -85.26) projected
  line L407 (592.1824, -85.26) -> (591.7819, -85.7819) projected
  line L408 (591.7819, -85.7819) -> (591.26, -86.1824) projected
  line L409 (591.26, -86.1824) -> (590.6522, -86.4341) projected
  line L410 (590.6522, -86.4341) -> (590, -86.52) projected
  line L411 (590, -86.52) -> (589.3478, -86.4341) projected
  line L412 (660, -164) -> (660, 0) projected
  line L413 (660, 0) -> (0, 0) projected
  line L414 (0, 0) -> (0, -164) projected
  line L415 (0, -164) -> (0.0398, -164.404) projected
  line L416 (0.0398, -164.404) -> (0.1577, -164.7926) projected
  line L417 (0.1577, -164.7926) -> (0.349, -165.1506) projected
  line L418 (0.349, -165.1506) -> (0.6066, -165.4645) projected
  line L419 (0.6066, -165.4645) -> (0.9204, -165.722) projected
  line L420 (0.9204, -165.722) -> (1.2785, -165.9134) projected
  line L421 (1.2785, -165.9134) -> (1.667, -166.0313) projected
  line L422 (1.667, -166.0313) -> (2.0711, -166.0711) projected
  line L423 (2.0711, -166.0711) -> (2.4751, -166.0313) projected
  line L424 (2.4751, -166.0313) -> (2.8636, -165.9134) projected
  line L425 (2.8636, -165.9134) -> (3.2217, -165.722) projected
  line L426 (3.2217, -165.722) -> (3.5355, -165.4645) projected
  line L427 (3.5355, -165.4645) -> (70, -99) projected
  line L428 (70, -99) -> (590, -99) projected
  line L429 (590, -99) -> (656.4645, -165.4645) projected
  line L430 (656.4645, -165.4645) -> (656.7783, -165.722) projected
  line L431 (656.7783, -165.722) -> (657.1364, -165.9134) projected
  line L432 (657.1364, -165.9134) -> (657.5249, -166.0313) projected
  line L433 (657.5249, -166.0313) -> (657.9289, -166.0711) projected
  line L434 (657.9289, -166.0711) -> (658.333, -166.0313) projected
  line L435 (658.333, -166.0313) -> (658.7215, -165.9134) projected
  line L436 (658.7215, -165.9134) -> (659.0796, -165.722) projected
  line L437 (659.0796, -165.722) -> (659.3934, -165.4645) projected
  line L438 (659.3934, -165.4645) -> (659.651, -165.1506) projected
  line L439 (659.651, -165.1506) -> (659.8423, -164.7926) projected
  line L440 (659.8423, -164.7926) -> (659.9602, -164.404) projected
  line L441 (659.9602, -164.404) -> (660, -164) projected
  point P0 (645, -139)
  point P1 (645, -84)
  point P2 (590, -84)
  point P3 (645, -14)
  point P4 (590, -14)
  point P5 (458.95, -14)
  point P6 (458.95, -84)
  point P7 (201.05, -14)
  point P8 (201.05, -84)
  point P9 (70, -84)
  point P10 (70, -14)
  point P11 (15, -14)
  point P12 (15, -84)
  point P13 (15, -139)
  point P14 (330, -84)
  point P15 (330, -14)
sketch "Sketch4" plane through (0, 0, 3) normal (0, 0, 1) x (1, 0, 0)
  line L0 (9.0091, -146.0565) -> (22.5386, -146.0565)
  line L1 (22.5386, -3.6524) -> (9.0091, -3.6524)
  line L2 (9.0091, -3.6524) -> (9.0091, -146.0565)
  line L3 (22.5386, -22.9148) -> (635.8099, -22.9148)
  line L4 (652.2603, -22.9148) -> (652.2603, -6.5692)
  line L5 (652.2603, -6.5692) -> (22.5386, -6.5692)
  line L6 (9.0091, -6.5692) -> (9.0091, -22.9148)
  line L7 (635.8099, -6.5692) -> (652.2603, -6.5692)
  line L8 (652.2603, -6.5692) -> (652.2603, -142.3663)
  line L9 (652.2603, -142.3663) -> (635.8099, -142.3663)
  line L10 (635.8099, -91.0795) -> (22.5386, -91.0795)
  line L11 (9.0091, -91.0795) -> (9.0091, -74.8545)
  line L12 (22.5386, -74.8545) -> (635.8099, -74.8545)
  line L13 (652.2603, -74.8545) -> (652.2603, -91.0795)
  line L14 (22.5386, -146.0565) -> (22.5386, -91.0795)
  line L15 (22.5386, -74.8545) -> (22.5386, -22.9148)
  line L16 (22.5386, -6.5692) -> (22.5386, -3.6524)
  line L17 (635.8099, -142.3663) -> (635.8099, -91.0795)
  line L18 (635.8099, -74.8545) -> (635.8099, -22.9148)
  point P0 (0, 0)
  constraints: 38 end point, 11 parallel, 6 perpendicular, 4 horizontal, 4 point on line, 1 midpoint
extrude "Extrusion2" add sketch "Sketch4" against normal up to surface (3 mm away)
sketch "Sketch5" plane through (0, 0, 3) normal (0, 0, 1) x (1, 0, 0)
  point P0 (0, 0)
hole "Hole1" at (15, -139, 3) at (15, -84, 3) at (15, -14, 3) at (70, -84, 3) at (70, -14, 3) at (201.05, -84, 3) at (201.05, -14, 3) at (458.95, -84, 3) at (458.95, -14, 3) at (590, -84, 3) at (645, -139, 3) at (590, -14, 3) at (645, -84, 3) at (645, -14, 3) at (330, -84, 3) at (330, -14, 3) direction (0, 0, -1) diameter 5 end through all